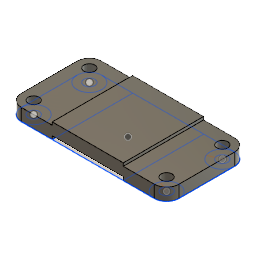
NOCTI Job 2 (Autodesk Fusion 360 design; units mm, degrees)
Autodesk Fusion 360 part; units mm, degrees
sketch "Sketch2" plane through (0, 0, 0) normal (0, 1, 0) x (1, 0, 0)
  circle A0 centre (-68.199, 28.575) radius 5.588
  circle A1 centre (-68.199, -28.575) radius 5.588
  circle A2 centre (68.199, -28.575) radius 5.588
  circle A3 centre (68.199, 28.575) radius 5.588
  circle A4 centre (68.199, 28.575) radius 12.7
  circle A5 centre (68.199, -28.575) radius 12.7
  circle A6 centre (-68.199, 28.575) radius 12.7
  circle A7 centre (-68.199, -28.575) radius 12.7
  line L0 (-80.899, 28.575) -> (-80.899, -28.575)
  line L1 (68.199, -41.275) -> (-68.199, -41.275)
  line L2 (80.899, 28.575) -> (80.899, -28.575)
  line L3 (68.199, 41.275) -> (-68.199, 41.275)
  line L4 (68.199, -28.575) -> (56.4856, -23.6672) construction
  line L5 (-36.449, 41.275) -> (-36.449, -41.275)
  line L6 (36.449, -41.275) -> (36.449, 41.275)
  line L7 (56.4856, 23.6672) -> (68.199, 28.575) construction
  dimension "d19" = 136.398
  dimension "d20" = 57.15
  dimension "d21" = 11.176
  dimension "d22" = 11.176
  dimension "d23" = 11.176
  dimension "d24" = 11.176
  dimension "d25" = 25.4
  dimension "d26" = 25.4
  dimension "d27" = 25.4
  dimension "d28" = 25.4
  measures "d21" diameter of A0
  measures "d22" diameter of A1
  measures "d23" diameter of A2
  measures "d24" diameter of A3
  measures "d25" diameter of A4
  measures "d26" diameter of A5
  measures "d27" diameter of A6
  measures "d28" diameter of A7
extrude "Extrude5" add sketch "Sketch2" along normal blind 15.748 contours L1 L3 L5 L6 makes body 1
extrude "Extrude4" add sketch "Sketch2" along normal blind 12.7 separate body contours A4 | A4 A5 L1 L2 L3 L6 | A5 | A6 A7 L0 L1 L3 L5 | A6 | A7 makes body 2 at (-45.4933, 0, 8.4757) makes body 3 at (45.4933, 0, 8.4757)
extrude "Extrude6" cut sketch "Sketch2" along normal blind 3.302 contours L1 L3 L5 L6 bodies 1
combine "Combine2" operation add target body 3 tool bodies 1 2
